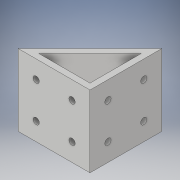
# Autodesk Inventor part: 15series_3inchCorner
Saved by Autodesk Inventor 2018 (Build 220112000, 112)
## iProperties
Created: 2020-03-10
Part Number: 15series_3inchCorner
Material: Generic
Document SubType Name: Modeling
Designer: natha
Density: 1 g/cm^3
Appearance: Default
Author: natha
Autodesk Inventor part; units mm, degrees
ref_plane "YZ Plane" through (0, 0, 0) normal (1, 0, 0) x (0, 1, 0)
ref_plane "XZ Plane" through (0, 0, 0) normal (0, 1, 0) x (-1, 0, 0)
ref_plane "XY Plane" through (0, 0, 0) normal (0, 0, 1) x (1, 0, 0)
sketch "Sketch1" plane through (0, 0, 0) normal (0, 1, 0) x (-1, 0, 0)
  line L0 (0, 0) -> (76.2, 0)
  line L1 (0, -76.2) -> (0, 0)
  line L2 (76.2, 0) -> (0, -76.2)
  line L3 (6.35, -6.35) -> (6.35, -58.8833)
  line L4 (58.982, -8.2377) -> (10.1183, -57.1015)
  line L5 (6.35, -6.35) -> (60.8697, -6.35)
  line L6 (60.8697, -6.35) -> (58.982, -8.2377)
  line L7 (6.35, -58.8833) -> (6.35, -60.8697)
  line L8 (6.35, -60.8697) -> (10.1183, -57.1015)
  dimension "d5" = 76.2
  dimension "d6" = 76.2
  dimension "d7" = 6.35
  dimension "d9" = 6.35
  constraints: 18 end point, 2 horizontal, 2 parallel, 1 collinear, 1 perpendicular, 1 point on line
  measures "d5" distance of L1.start L0.start
  measures "d6" distance of L0.start L0.end
  measures "d7" distance between parallel lines of L1 L3
  measures "d9" distance between parallel lines of L4 L2
extrude "Extrusion1" add sketch "Sketch1" along normal blind 76.2
sketch "Sketch2" plane through (0, 0, 0) normal (1, 0, 0) x (0, 0, -1)
  circle A0 centre (19.05, 19.05) radius 3.3274
  circle A1 centre (57.15, 19.05) radius 3.3274
  circle A2 centre (57.15, 57.15) radius 3.3274
  circle A3 centre (19.05, 57.15) radius 3.3274
  line L0 (0, 76.2) -> (76.2, 76.2) projected
  line L1 (76.2, 0) -> (76.2, 76.2) projected
  line L2 (76.2, 0) -> (0, 0) projected
  line L3 (0, 0) -> (0, 76.2) projected
  dimension "d12" = 6.6548
  dimension "d13" = 6.6548
  dimension "d14" = 6.6548
  dimension "d15" = 6.6548
  dimension "d16" = 19.05
  dimension "d17" = 19.05
  dimension "d18" = 19.05
  dimension "d19" = 19.05
  dimension "d20" = 19.05
  dimension "d21" = 19.05
  dimension "d22" = 19.05
  dimension "d23" = 19.05
  constraints: 4 centre point
  measures "d12" diameter of A0
  measures "d13" diameter of A1
  measures "d14" diameter of A2
  measures "d15" diameter of A3
  measures "d16" distance from line of L0 A2.centre
  measures "d17" distance from line of L1 A2.centre
  measures "d18" distance from line of L1 A1.centre
  measures "d19" distance from line of L2 A1.centre
  measures "d20" distance from line of L2 A0.centre
  measures "d21" distance from line of L3 A0.centre
  measures "d22" distance from line of L0 A3.centre
  measures "d23" distance from line of L3 A3.centre
extrude "Extrusion2" cut sketch "Sketch2" against normal blind 25.4 contours A0 | A1 | A2 | A3
sketch "Sketch3" plane through (-76.2, 0, 0) normal (0, 0, 1) x (1, 0, 0)
  circle A0 centre (57.15, 19.05) radius 3.3274
  circle A1 centre (19.05, 19.05) radius 3.3274
  circle A2 centre (19.05, 57.15) radius 3.3274
  circle A3 centre (57.15, 57.15) radius 3.3274
  line L0 (76.2, 0) -> (0, 0) projected
  line L1 (76.2, 0) -> (76.2, 76.2) projected
  line L2 (0, 76.2) -> (76.2, 76.2) projected
  line L3 (0, 0) -> (0, 76.2) projected
  dimension "d26" = 6.6548
  dimension "d27" = 6.6548
  dimension "d28" = 6.6548
  dimension "d29" = 6.6548
  dimension "d30" = 19.05
  dimension "d31" = 19.05
  dimension "d32" = 19.05
  dimension "d33" = 19.05
  dimension "d34" = 19.05
  dimension "d35" = 19.05
  dimension "d36" = 19.05
  dimension "d37" = 19.05
  constraints: 4 centre point
  measures "d26" diameter of A0
  measures "d27" diameter of A1
  measures "d28" diameter of A2
  measures "d29" diameter of A3
  measures "d30" distance from line of L0 A0.centre
  measures "d31" distance from line of L1 A0.centre
  measures "d32" distance from line of L1 A3.centre
  measures "d33" distance from line of L2 A3.centre
  measures "d34" distance from line of L3 A2.centre
  measures "d35" distance from line of L2 A2.centre
  measures "d36" distance from line of L0 A1.centre
  measures "d37" distance from line of L3 A1.centre
extrude "Extrusion3" cut sketch "Sketch3" against normal blind 25.4 contours A0 | A1 | A2 | A3
body "Solid1"
